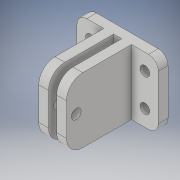
# Autodesk Inventor part: pleksi_mocowanie
Saved by Autodesk Inventor 2019 (Build 230136000, 136)
## iProperties
Created: 2018-10-16
Part Number: pleksi_mocowanie
Material: Ogólny
Document SubType Name: Modeling
Designer: user
Density: 1 g/cm^3
Appearance: Domyślna
Author: user
Autodesk Inventor part; units mm, degrees
ref_plane "YZ Plane" through (0, 0, 0) normal (1, 0, 0) x (0, 1, 0)
ref_plane "XZ Plane" through (0, 0, 0) normal (0, 1, 0) x (-1, 0, 0)
ref_plane "XY Plane" through (0, 0, 0) normal (0, 0, 1) x (1, 0, 0)
sketch "Szkic1" plane through (0, 0, 0) normal (0, 0, 1) x (1, 0, 0)
  line L0 (-12.5, -10) -> (12.5, -10)
  line L1 (12.5, -10) -> (12.5, 10)
  line L2 (12.5, 10) -> (-12.5, 10)
  line L3 (-12.5, 10) -> (-12.5, -10)
  line L4 (-12.5, -10) -> (12.5, 10) construction
  line L5 (12.5, -10) -> (-12.5, 10) construction
  point P0 (0, 0)
  dimension "d0" = 25
  dimension "d1" = 20
  constraints: 12 end point, 2 midpoint, 2 parallel, 1 horizontal, 1 perpendicular
  measures "d0" distance of L2.end L1.end
  measures "d1" distance of L1.end L0.end
extrude "Wyciągnięcie proste1" add sketch "Szkic1" along normal blind 3
sketch "Szkic2" plane through (0, 0, 3) normal (0, 0, 1) x (1, 0, 0)
  line L0 (1.25, -10) -> (4.25, -10)
  line L1 (4.25, -10) -> (4.25, 10)
  line L2 (4.25, 10) -> (1.25, 10)
  line L3 (1.25, 10) -> (1.25, -10)
  line L4 (1.25, -10) -> (4.25, 10) construction
  line L5 (4.25, -10) -> (1.25, 10) construction
  line L6 (-12.5, -10) -> (12.5, -10) projected
  line L7 (12.5, 10) -> (-12.5, 10) projected
  line L8 (0, 10) -> (0, -10) construction
  line L9 (-1.25, -10) -> (-4.25, -10)
  line L10 (-4.25, -10) -> (-4.25, 10)
  line L11 (-4.25, 10) -> (-1.25, 10)
  line L12 (-1.25, 10) -> (-1.25, -10)
  line L13 (-1.25, -10) -> (-4.25, 10) construction
  line L14 (-4.25, -10) -> (-1.25, 10) construction
  point P0 (0, 0)
  point P1 (2.75, 0)
  point P2 (-2.75, 0)
  dimension "d4" = 3
  dimension "d5" = 20
  dimension "d6" = 2.75
  dimension "d7" = 10
  constraints: 26 end point, 6 midpoint, 5 symmetric about line, 2 parallel, 1 horizontal, 1 perpendicular
  measures "d4" distance of L2.end L1.end
  measures "d5" distance of L1.end L0.end
  measures "d6" distance of point (0, 0) point (2.75, 0)
  measures "d7" distance from line of L6 point (2.75, 0)
extrude "Wyciągnięcie proste2" add sketch "Szkic2" along normal blind 20 contours L3 L2 L1 L0 | L6 L10 L7 L12
sketch "Szkic3" plane through (4.25, -10, 3) normal (1, 0, 0) x (0, 0, -1)
  line L0 (-20, 0) -> (-20, 20) projected
  line L1 (0, 20) -> (-20, 20) projected
  point P0 (3, 10)
  point P1 (-17, 10)
  dimension "d10" = 3
  dimension "d11" = 10
  measures "d10" distance from line of L0 point (-17, 10)
  measures "d11" distance from line of L1 point (-17, 10)
hole "Otwór1" at (4.25, 0, 20) direction (-1, 0, 0) diameter 3 end through all
fillet "Zaokrąglenie1" radius 5 4 edges at (2.75, -10, 23) (-2.75, -10, 23) (-2.75, 10, 23) (2.75, 10, 23)
fillet "Zaokrąglenie2" radius 3 4 edges at (12.5, 10, 1.5) (12.5, -10, 1.5) (-12.5, -10, 1.5) (-12.5, 10, 1.5)
sketch "Szkic4" plane through (0, 0, 3) normal (0, 0, 1) x (1, 0, 0)
  line L0 (-12.5, 7) -> (-12.5, -7) projected
  line L1 (-9.5, -10) -> (-4.25, -10) projected
  line L2 (-1.25, -10) -> (1.25, -10) projected
  line L3 (0, -10) -> (0, 10) construction
  line L4 (1.25, 10) -> (-1.25, 10) projected
  line L5 (12.5, -7) -> (12.5, 7) projected
  line L6 (12.5, 0) -> (-12.5, 0) construction
  point P0 (0, 0)
  point P1 (-8.375, -5)
  point P2 (8.375, -5)
  point P3 (-8.375, 5)
  point P4 (8.375, 5)
  dimension "d21" = 4.125
  dimension "d22" = 5
  constraints: 4 end point, 4 midpoint, 3 symmetric about line
  measures "d21" distance from line of L0 point (-8.375, -5)
  measures "d22" distance from line of L1 point (-8.375, -5)
hole "Otwór2" at (-8.375, -5, 3) at (8.375, -5, 3) at (8.375, 5, 3) at (-8.375, 5, 3) direction (0, 0, -1) diameter 3 end through all
